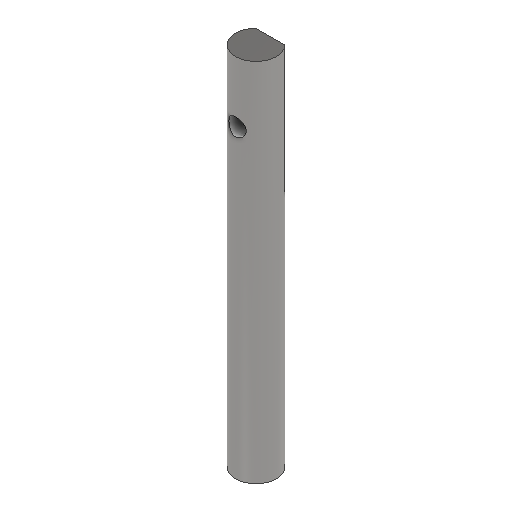
# Autodesk Inventor part: Rotary_Feedthorough_top
Saved by Autodesk Inventor 2026.2 (Build 302298000, 298)
## iProperties
Created: 2026-05-26
Part Number: Rotary_Feedthorough_top
Material: Generic
Document SubType Name: Modeling
Designer: zetsu
Density: 1 g/cm^3
Appearance: Default
Author: zetsu
Autodesk Inventor part; units mm, degrees
ref_plane "YZ Plane" through (0, 0, 0) normal (1, 0, 0) x (0, 1, 0)
ref_plane "XZ Plane" through (0, 0, 0) normal (0, 1, 0) x (-1, 0, 0)
ref_plane "XY Plane" through (0, 0, 0) normal (0, 0, 1) x (1, 0, 0)
sketch "スケッチ2" plane through (0, 0, 0) normal (0, 1, 0) x (-1, 0, 0)
  circle A0 centre (0, 0) radius 4
  dimension "d0" = 8
  constraints: 1 centre point, 1 coincident
  measures "d0" diameter of A0
extrude "押し出し1" add sketch "スケッチ2" along normal blind 72
sketch "スケッチ3" plane through (0, 72, 0) normal (0, 1, 0) x (1, 0, 0)
  line L0 (-4.1769, 6.014) -> (4.0611, 6.014)
  line L1 (4.0611, 6.014) -> (4.0611, 2.8)
  line L2 (4.0611, 2.8) -> (-4.1769, 2.8)
  line L3 (-4.1769, 2.8) -> (-4.1769, 6.014)
  point P0 (0, 0)
  dimension "d3" = 2.8
  constraints: 8 end point, 2 parallel, 1 horizontal, 1 perpendicular
  measures "d3" distance from line of point (0, 0) L2
extrude "押し出し2" cut sketch "スケッチ3" against normal blind 25
sketch "スケッチ4" plane through (2.8566, 72, -2.8) normal (0, 0, -1) x (-1, 0, 0)
  line L0 (6.8566, 0) -> (-1.1434, 0) projected
  line L1 (2.8566, 0) -> (2.8566, -27.2038) construction
  circle A0 centre (2.8566, -12) radius 1.7
  point P0 (2.8566, -72)
  point P1 (5.7131, 0)
  point P2 (0, 0)
  dimension "d6" = 3.4
  dimension "d7" = 12
  constraints: 2 end point, 1 centre point, 1 midpoint, 1 point on line, 1 vertical
  measures "d6" diameter of A0
  measures "d7" distance from line of L0 A0.centre
extrude "押し出し3" cut sketch "スケッチ4" against normal through all
